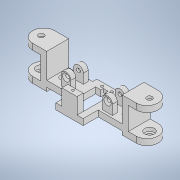
# Autodesk Inventor part: Основа рулевого механизма_backup
Saved by Autodesk Inventor 2020 (Build 240168000, 168)
## iProperties
Created: 2021-03-14
Part Number: Основа рулевого механизма_backup
Material: Типовые
Document SubType Name: Обычные детали
Designer: Антон
Density: 1 g/cm^3
Appearance: По умолчанию
Mass: 18.7306 g
Surface Area: 112.354 cm^2
Volume: 18.7306 cm^3
Sheet Metal Rule: По умолчанию
Author: Антон
Autodesk Inventor part; units mm, degrees
ref_plane "YZ Plane" through (0, 0, 0) normal (1, 0, 0) x (0, 1, 0)
sketch "Эскиз1" plane through (0, 0, 0) normal (0, 0, 1) x (1, 0, 0)
  line L0 (0, 0) -> (-20.5, 0)
  line L1 (-20.5, 0) -> (-20.5, 28.6)
  line L2 (-20.5, 28.6) -> (0, 28.6)
  line L3 (0, 28.6) -> (0, 0)
  line L4 (-20.5, 0) -> (-20.5, 5)
  line L5 (-20.5, 5) -> (-5, 5)
  line L6 (-5, 5) -> (-5, 23.6)
  line L7 (-5, 23.6) -> (-20.5, 23.6)
  line L8 (-20.5, 23.6) -> (-20.5, 5)
  point P0 (-20.5, 23.6)
  point P1 (0, 3)
  dimension "d8" = 20.5
  dimension "d9" = 28.6
  dimension "d10" = 5
  dimension "d11" = 15.5
  dimension "d12" = 18.6
  constraints: 18 end point, 4 parallel, 2 horizontal, 2 perpendicular, 2 point on line
  measures "d8" distance of L1.end L2.end
  measures "d9" distance of L0.end L1.end
  measures "d10" distance of L0.end L4.end
  measures "d11" distance of L7.end L6.end
  measures "d12" distance of L6.end L5.end
extrude "Выдавливание1" add sketch "Эскиз1" along normal blind 18 contours L0 L1 L5 L6 L7 L2 L3
sketch "Эскиз4" plane through (-20.5, 23.6, 0) normal (0, -1, 0) x (1, 0, 0)
  line L0 (0, 0) -> (0, 18) projected
  line L1 (0, 9) -> (7, 9)
  circle A0 centre (7, 9) radius 4
  point P0 (20.5, 0)
  dimension "d31" = 7
  dimension "d32" = 8
  constraints: 2 end point, 1 centre point, 1 coincident, 1 horizontal, 1 midpoint
  measures "d31" distance of L1.start L1.end
  measures "d32" diameter of A0
extrude "Выдавливание2" cut sketch "Эскиз4" against normal blind 3
sketch "Эскиз5" plane through (-20.5, 5, 0) normal (0, 1, 0) x (1, 0, 0)
  circle A0 centre (7, -9) radius 4 projected
  point P0 (20.5, 0)
extrude "Выдавливание3" cut sketch "Эскиз5" against normal blind 3
fillet "Сопряжение1" radius 9 4 edges at (-20.5, 26.1, 18) (-20.5, 26.1, 0) (-20.5, 2.5, 18) (-20.5, 2.5, 0)
sketch "Эскиз6" plane through (0, 28.6, 18) normal (0, 1, 0) x (1, 0, 0)
  circle A0 centre (-13.5, 9) radius 4 projected
  point P0 (0, 18)
hole "Отверстие2" at (-13.5, 28.6, 9) direction (0, -1, 0) diameter 4.5 end through all
ref_plane "РабПлоскость7" through (0, 3, 0) normal (0, -1, 0) x (1, 0, 0)
sketch "Эскиз36" plane through (0, 3, 0) normal (0, -1, 0) x (1, 0, 0)
  line L0 (0, 0) -> (-11.5, 0) projected
  line L1 (0, 0) -> (31.05, 0)
  line L2 (31.05, 0) -> (31.05, 18)
  line L3 (31.05, 18) -> (0, 18)
  line L4 (0, 18) -> (0, 0)
  line L5 (-11.5, 18) -> (0, 18) projected
  dimension "d217" = 31.05
  constraints: 8 end point, 2 parallel, 1 collinear, 1 horizontal, 1 perpendicular
  measures "d217" distance of L3.end L2.end
extrude "Выдавливание23" add sketch "Эскиз36" against normal blind 5 from surface at 0
mirror "Зеркальное отражение6" about plane through (31.05, 3, 18) normal (1, 0, 0)
ref_plane "РабПлоскость6" through (31.05, 28.6, 18) normal (1, 0, 0) x (0, 0, -1)
sketch "Эскиз43" plane through (0, 0, 0) normal (0, 0, -1) x (-1, 0, 0)
  line L0 (-42.3, 8) -> (-19.8, 8)
  line L1 (-19.8, 8) -> (-19.8, 3)
  line L2 (-19.8, 3) -> (-42.3, 3)
  line L3 (-42.3, 3) -> (-42.3, 8)
  line L4 (-62.1, 8) -> (0, 8) projected
  line L5 (-62.1, 3) -> (0, 3) projected
  point P0 (-89.6, 0)
  point P1 (-31.05, 8)
  dimension "d260" = 22.5
  constraints: 8 end point, 2 collinear, 2 midpoint, 2 parallel, 1 horizontal, 1 perpendicular
  measures "d260" distance between parallel lines of L1 L3
extrude "Выдавливание27" add sketch "Эскиз43" along normal blind 3.45
sketch "Эскиз46" plane through (0, 0, 18) normal (0, 0, 1) x (1, 0, 0)
  line L0 (19.8, 3) -> (19.8, 8) projected
  line L1 (19.8, 8) -> (42.3, 8) projected
  line L2 (42.3, 8) -> (42.3, 3) projected
  line L3 (42.3, 3) -> (19.8, 3) projected
  point P0 (0, 0)
extrude "Выдавливание29" add sketch "Эскиз46" along normal blind 12.35
sketch "Эскиз48" plane through (0, 8, 18) normal (0, 1, 0) x (1, 0, 0)
  line L0 (37.3, -7.35) -> (24.8, -7.35)
  line L1 (24.8, -7.35) -> (24.8, 15.45)
  line L2 (24.8, 15.45) -> (37.3, 15.45)
  line L3 (37.3, 15.45) -> (37.3, -7.35)
  line L4 (42.3, 0) -> (42.3, -12.35) projected
  line L5 (19.8, 0) -> (19.8, -12.35) projected
  line L6 (42.3, 0) -> (19.8, 0)
  line L7 (31.05, -7.35) -> (31.05, 0)
  point P0 (0, 18)
  dimension "d280" = 12.5
  dimension "d281" = 22.8
  dimension "d295" = 7.35
  constraints: 12 end point, 2 horizontal, 2 midpoint, 2 parallel, 2 perpendicular
  measures "d280" distance of L1.end L2.end
  measures "d281" distance of L0.end L1.end
  measures "d295" distance of L7.start L7.end
extrude "Выдавливание31" cut sketch "Эскиз48" against normal through all
sketch "Эскиз47" plane through (0, 8, 18) normal (0, 1, 0) x (1, 0, 0)
  line L0 (24.8, -12.35) -> (37.3, -12.35)
  line L1 (37.3, -12.35) -> (37.3, -7.35)
  line L2 (37.3, -7.35) -> (24.8, -7.35)
  line L3 (24.8, -7.35) -> (24.8, -12.35)
  line L4 (42.3, -12.35) -> (19.8, -12.35) projected
  line L5 (37.3, -7.35) -> (24.8, -7.35) projected
  line L6 (24.8, -7.35) -> (24.8, 15.45) projected
  point P0 (0, 18)
  point P1 (31.05, -7.35)
  constraints: 8 end point, 2 collinear, 2 midpoint, 2 parallel, 1 horizontal, 1 perpendicular
extrude "Выдавливание30" add sketch "Эскиз47" along normal blind 13.15
sketch "Эскиз50" plane through (0, 21.15, 18) normal (0, 1, 0) x (1, 0, 0)
  line L0 (31.05, -7.35) -> (31.05, -9.425)
  line L1 (37.3, -7.35) -> (24.8, -7.35) projected
  point P0 (0, 18)
  dimension "d285" = 2.075
  constraints: 2 end point, 1 midpoint, 1 vertical
  measures "d285" distance of L0.start L0.end
hole "Отверстие13" at (31.05, 21.15, 27.425) direction (0, -1, 0) diameter 2 depth 5 tip angle 118
sketch "Эскиз51" plane through (-11.5, 3, 9) normal (0, -1, 0) x (1, 0, 0)
  line L0 (48.8, -6.45) -> (36.3, -6.45) projected
  line L1 (36.3, -6.45) -> (38.55, -6.45)
  line L2 (48.8, -6.45) -> (46.55, -6.45)
  line L3 (38.55, -6.45) -> (38.55, -9.45)
  line L4 (46.55, -6.45) -> (46.55, -9.45)
  dimension "d347" = 8
  dimension "d348" = 3
  constraints: 8 end point, 2 collinear, 2 equal length, 2 perpendicular, 1 vertical
  measures "d347" distance between parallel lines of L4 L3
  measures "d348" distance of L1.end L3.end
hole "Отверстие14" at (27.05, 3, -0.45) at (35.05, 3, -0.45) direction (0, 1, 0) diameter 2.2 end through all countersink diameter 3.9 countersink angle 90
sketch "Эскиз52" plane through (0, 8, 18) normal (0, 1, 0) x (1, 0, 0)
  line L0 (33.05, 15.45) -> (29.05, 15.45)
  line L1 (29.05, 15.45) -> (29.05, 17.45)
  line L2 (29.05, 17.45) -> (33.05, 17.45)
  line L3 (33.05, 17.45) -> (33.05, 15.45)
  line L4 (24.8, 15.45) -> (37.3, 15.45) projected
  point P0 (0, 18)
  point P1 (31.05, 15.45)
  dimension "d305" = 4
  dimension "d306" = 2
  constraints: 8 end point, 2 midpoint, 2 parallel, 1 horizontal, 1 perpendicular
  measures "d305" distance of L1.end L2.end
  measures "d306" distance of L0.end L1.end
extrude "Выдавливание32" cut sketch "Эскиз52" against normal through all
sketch "Эскиз53" plane through (29.05, 8, 0.55) normal (0, 0, 1) x (1, 0, 0)
  line L0 (4, -5) -> (0, -5) projected
  line L1 (0, -5) -> (4, -5)
  line L2 (4, -5) -> (4, -3)
  line L3 (4, -3) -> (0, -3)
  line L4 (0, -3) -> (0, -5)
  line L5 (4, 0) -> (4, -5) projected
  point P0 (-29.05, -8)
  dimension "d349" = 2
  constraints: 8 end point, 2 parallel, 1 collinear, 1 horizontal, 1 perpendicular
  measures "d349" distance between parallel lines of L0 L3
extrude "Выдавливание33" cut sketch "Эскиз53" against normal through all
sketch "Эскиз54" plane through (0, 8, 18) normal (0, 1, 0) x (1, 0, 0)
  line L0 (0, 18) -> (0, 0) projected
  line L1 (0, 9) -> (5, 9)
  dimension "d312" = 5
  constraints: 2 end point, 1 horizontal, 1 midpoint
  measures "d312" distance of L1.start L1.end
hole "Отверстие15" at (5, 8, 9) direction (0, -1, 0) diameter 3.2 end through all countersink diameter 6 countersink angle 90
sketch "Эскиз56" plane through (0, 8, 18) normal (0, 1, 0) x (1, 0, 0)
  line L0 (-11.5, 18) -> (0, 18) projected
  line L1 (10, 16.1) -> (18, 16.1)
  line L2 (18, 16.1) -> (18, 12.1)
  line L3 (18, 12.1) -> (10, 12.1)
  line L4 (10, 12.1) -> (10, 16.1)
  line L5 (10, 5.9) -> (18, 5.9)
  line L6 (18, 5.9) -> (18, 1.9)
  line L7 (18, 1.9) -> (10, 1.9)
  line L8 (10, 1.9) -> (10, 5.9)
  line L9 (14, 16.1) -> (14, 18)
  line L10 (14, 1.9) -> (14, 0)
  line L11 (19.8, 0) -> (0, 0) projected
  line L12 (19.8, 18) -> (0, 18) projected
  line L13 (0, 18) -> (0, 0) projected
  point P0 (27.8, 18)
  dimension "d328" = 8
  dimension "d329" = 4
  dimension "d330" = 6.2
  dimension "d331" = 10
  constraints: 20 end point, 4 collinear, 4 parallel, 4 perpendicular, 2 horizontal, 2 midpoint, 2 point on line, 1 vertical
  measures "d328" distance of L1.start L1.end
  measures "d329" distance of L3.end L1.start
  measures "d330" distance between parallel lines of L5 L3
  measures "d331" distance between parallel lines of L13 L8
extrude "Выдавливание34" add sketch "Эскиз56" along normal blind 12
fillet "Сопряжение6" radius 4 4 edges at (18, 20, 14.1) (18, 20, 3.9) (10, 20, 3.9) (10, 20, 14.1)
sketch "Эскиз57" plane through (10, 8, 16.1) normal (0, 0, 1) x (1, 0, 0)
  line L0 (8, 0) -> (0, 0) projected
  line L1 (9.8, 0) -> (-10, 0) projected
  line L2 (0, 0) -> (8, 0) projected
  arc A0 (8, 8) -> (0, 8) centre (4, 8) ccw projected
  point P0 (-10, -8)
hole "Отверстие16" at (14, 16, 16.1) direction (0, 0, -1) diameter 3.2 end through all countersink diameter 6 countersink angle 90
sketch "Эскиз58" plane through (18, 8, 1.9) normal (0, 0, -1) x (-1, 0, 0)
  circle A0 centre (4, 8) radius 1.6 projected
  line L0 (6.8, 6.3834) -> (4, 4.7668)
  line L1 (4, 4.7668) -> (1.2, 6.3834)
  line L2 (1.2, 6.3834) -> (1.2, 9.6166)
  line L3 (1.2, 9.6166) -> (4, 11.2332)
  line L4 (4, 11.2332) -> (6.8, 9.6166)
  line L5 (6.8, 9.6166) -> (6.8, 6.3834)
  line L6 (8, 0) -> (8, 8) projected
  point P0 (18, -8)
  dimension "d352" = 5.6
  constraints: 12 end point, 1 coincident, 1 parallel, 13 other
  measures "d352" distance between parallel lines of L2 L5
extrude "Выдавливание35" cut sketch "Эскиз58" against normal blind 2.6 contours A0 | L0 L1 L2 L3 L4 L5
mirror "Зеркальное отражение8" about plane through (31.05, 28.6, 18) normal (1, 0, 0) of "Отверстие15", "Выдавливание35", "Отверстие16", "Сопряжение6", "Выдавливание34"
equation "\"d10\" = -0.5 * d12 + 0.5 * d9"
